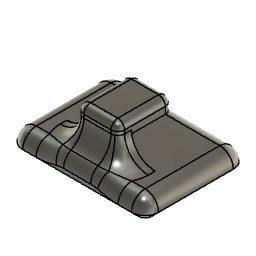
hook v1 (Autodesk Fusion 360 design; units mm, degrees)
Autodesk Fusion 360 part; units mm, degrees
sketch "Sketch1" plane through (0, 0, 0) normal (0, 0, 1) x (1, 0, 0)
sketch "Sketch2" plane through (0, 0, 0) normal (0, 0, 1) x (1, 0, 0)
  line L0 (0, 15) -> (20, 15)
  line L1 (20, 15) -> (20, 0)
  line L2 (20, 0) -> (0, 0)
  line L3 (0, 0) -> (0, 15)
  line L4 (7, 11) -> (13, 11)
  line L5 (13, 11) -> (13, 3)
  line L6 (13, 3) -> (7, 3)
  line L7 (7, 3) -> (7, 11)
  line L8 (7, 5) -> (13, 5)
  line L9 (13, 5) -> (13, 3)
  line L10 (13, 3) -> (7, 3)
  line L11 (7, 3) -> (7, 5)
  constraint horizontal L0
  constraint vertical L1
  constraint horizontal L2
  constraint vertical L3
  constraint horizontal L4
  constraint vertical L5
  constraint horizontal L6
  constraint vertical L7
  constraint horizontal L8
  constraint vertical L9
  constraint horizontal L10
  constraint vertical L11
  constraint coincident L7 L8.start
extrude "Extrude1" add sketch "Sketch2" along normal blind 3 contours L0 L1 L2 L3 | L4 L5 L7 L8 | L5 L6 L7 L8 L9 L10 L11 makes body 1
extrude "Extrude2" add sketch "Sketch2" along normal blind 5 separate body contours L5 L6 L7 L8 L9 L10 L11 makes body 2
extrude "Extrude3" add 1 faces at (9, 4.3333, 5) along direction (0, 0, 1) blind 3 on bodies 2 bodies 2
sketch "Sketch3" plane through (7, 0, 0) normal (-1, 0, 0) x (0, -1, 0)
  line L0 (-5, 0) -> (-3, 0)
  line L1 (-3, 0) -> (-3, 8)
  line L2 (-3, 8) -> (-5, 8)
  line L3 (-5, 8) -> (-5, 0)
sketch "Sketch4" plane through (0, 3, 0) normal (0, -1, 0) x (1, 0, 0)
  line L0 (7, 0) -> (13, 0)
  line L1 (13, 0) -> (13, 8)
  line L2 (13, 8) -> (7, 8)
  line L3 (7, 8) -> (7, 0)
  line L4 (7, 6) -> (13, 6)
  constraint coincident L3 L4.start
  constraint coincident L1 L4.end
  constraint perpendicular L1 L4
extrude "Extrude4" add sketch "Sketch4" against normal blind 8 separate body contours L1 L2 L3 L4 makes body 3
fillet "Fillet1" radius 2 4 edges at (0, 15, 1.5) (0, 0, 1.5) (20, 0, 1.5) (20, 15, 1.5) on bodies 1
fillet "Fillet2" radius 1 4 edges at (13, 3, 7) (13, 11, 7) (7, 3, 7) (7, 11, 7) on bodies 3
fillet "Fillet3" radius 1 1 edges at (13, 3, 4) on bodies 2
fillet "Fillet4" radius 1 1 edges at (7, 3, 4) on bodies 2
fillet "Fillet5" radius 1 5 edges at (7, 4.5, 8) (7.2929, 3.2929, 8) (10, 3, 8) (12.7071, 3.2929, 8) (13, 4.5, 8) on bodies 2
combine "Combine1" operation add target body 3 tool bodies 2 1
fillet "Fillet6" radius 3.5 5 edges at (7, 4.5, 3) (7.2929, 3.2929, 3) (10, 3, 3) (12.7071, 3.2929, 3) (13, 4.5, 3) on bodies 3
fillet "Fillet7" radius 1 8 edges at (12.7071, 10.7071, 8) (10, 11, 8) (7.2929, 10.7071, 8) (7, 7, 8) (7.2929, 3.2929, 8) (10, 3, 8) (12.7071, 3.2929, 8) (13, 7, 8) on bodies 3
fillet "Fillet8" radius 2 12 edges at (19.4142, 14.4142, 3) (10, 15, 3) (0.5858, 14.4142, 3) (0, 7.5, 3) (0.5858, 0.5858, 3) (3.9692, 0, 3) (6.9613, 0, 3.0189) (10, 0, 3.0359) (13.0387, 0, 3.0189) (16.0308, 0, 3) (19.4142, 0.5858, 3) (20, 7.5, 3) on bodies 3
chamfer "Chamfer1" distance 1 angle 45 8 edges at (10, 15, 0) (19.4142, 14.4142, 0) (20, 7.5, 0) (19.4142, 0.5858, 0) (10, 0, 0) (0.5858, 0.5858, 0) (0, 7.5, 0) (0.5858, 14.4142, 0) on bodies 3
